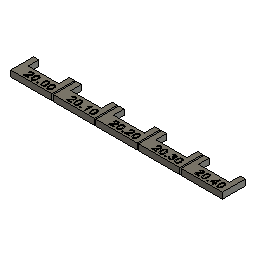
tolerance tester sloted v2 (Autodesk Fusion 360 design; units mm, degrees)
Autodesk Fusion 360 part; units mm, degrees
note: some values were not read from the file. Set by a fixed rule: which sketch regions a step uses.
sketch "Sketch1" plane through (0, 0, 0) normal (0, 1, 0) x (1, 0, 0)
  line L0 (0, 0) -> (27, 0)
  line L1 (27, 0) -> (27, -8)
  line L2 (27, -8) -> (0, -8)
  line L3 (0, -8) -> (0, 0)
  line L4 (27, 0) -> (0, 0)
  line L5 (0, 0) -> (0, 7)
  line L6 (27, 7) -> (27, 0)
  line L7 (13.5, 0) -> (13.5, 3.5)
  line L8 (3.5, 7) -> (3.5, 0)
  line L9 (3.5, 0) -> (23.5, 0)
  line L10 (23.5, 0) -> (23.5, 7)
  line L11 (23.5, 7) -> (3.5, 0) construction
  line L12 (3.5, 7) -> (23.5, 0) construction
  line L13 (0, 7) -> (3.5, 7)
  line L14 (23.5, 7) -> (27, 7)
  line L15 (51.5, 0) -> (51.4999, 7)
  line L16 (31.4, 0) -> (51.5, 0)
  line L17 (31.3999, 7) -> (31.4, 0)
  line L18 (27.9499, 0) -> (27.9499, 7)
  line L19 (27.9499, -8) -> (27.9499, 0)
  line L20 (27.9499, 0) -> (54.9499, 0)
  line L21 (54.9499, -8) -> (27.9499, -8)
  line L22 (54.9499, 0) -> (54.9499, -8)
  line L23 (27.9499, 7) -> (31.3999, 7)
  line L24 (54.9499, 7) -> (54.9499, 0)
  line L25 (54.9499, 0) -> (27.9499, 0)
  line L26 (51.4999, 7) -> (54.9499, 7)
  line L27 (55.8999, 7) -> (59.2999, 7)
  line L28 (107.5, 7) -> (110.85, 7)
  line L29 (55.8999, 0) -> (82.8999, 0)
  line L30 (79.4999, 0) -> (79.4999, 7)
  line L31 (83.85, -8) -> (83.85, 0)
  line L32 (59.2999, 0) -> (79.4999, 0)
  line L33 (59.2999, 7) -> (79.4999, 0) construction
  line L34 (59.2999, 7) -> (59.2999, 0)
  line L35 (69.3999, 0) -> (69.3999, 3.5)
  line L36 (79.4999, 7) -> (82.8999, 7)
  line L37 (82.8999, 0) -> (82.8999, -8)
  line L38 (107.5, 0) -> (107.5, 7)
  line L39 (87.2, 7) -> (87.2, 0)
  line L40 (55.8999, -8) -> (55.8999, 0)
  line L41 (87.2, 0) -> (107.5, 0)
  line L42 (110.85, 7) -> (110.85, 0)
  line L43 (82.8999, 0) -> (55.8999, 0)
  line L44 (107.5, 7) -> (87.2, 0) construction
  line L45 (83.85, 7) -> (87.2, 7)
  line L46 (110.85, 0) -> (83.85, 0)
  line L47 (110.85, -8) -> (83.85, -8)
  line L48 (83.85, 0) -> (83.85, 7)
  line L49 (79.4999, 7) -> (59.2999, 0) construction
  line L50 (82.8999, 7) -> (82.8999, 0)
  line L51 (97.35, 0) -> (97.35, 3.5)
  line L52 (55.8999, 0) -> (55.8999, 7)
  line L53 (83.85, 0) -> (110.85, 0)
  line L54 (110.85, 0) -> (110.85, -8)
  line L55 (87.2, 7) -> (107.5, 0) construction
  line L56 (82.8999, -8) -> (55.8999, -8)
  line L57 (7.0081, -6.0164) -> (18.0049, -5.9962) construction
  line L58 (18.0049, -5.9962) -> (17.9975, -1.9799) construction
  line L59 (17.9975, -1.9799) -> (7.0007, -2.0001) construction
  line L60 (7.0007, -2.0001) -> (7.0081, -6.0164) construction
  line L61 (7.0007, -2.0001) -> (135.5, -2.0001)
  line L62 (7.0081, -6.0164) -> (114.0079, -5.8204)
  line L63 (27.9499, -2.0001) -> (34.9499, -2.0001)
  line L64 (34.9499, -2.0001) -> (45.9489, -2.0001)
  line L65 (34.9544, -5.9574) -> (45.9521, -5.9451) construction
  line L66 (45.9521, -5.9451) -> (45.9477, -1.9877) construction
  line L67 (45.9477, -1.9877) -> (34.9499, -2.0001) construction
  line L68 (34.9499, -2.0001) -> (34.9544, -5.9574) construction
  line L69 (55.8999, -2.0001) -> (62.8999, -2.0001)
  line L70 (62.8999, -2.0001) -> (73.8899, -2.0001)
  line L71 (62.9041, -5.9057) -> (73.8932, -5.8939) construction
  line L72 (73.8932, -5.8939) -> (73.889, -1.9883) construction
  line L73 (73.889, -1.9883) -> (62.8999, -2.0001) construction
  line L74 (62.8999, -2.0001) -> (62.9041, -5.9057) construction
  line L75 (138.8, 0) -> (111.8, 0)
  line L76 (115.1, 0) -> (135.5, 0)
  line L77 (138.8, 7) -> (138.8, 0)
  line L78 (138.8, 0) -> (138.8, -8)
  line L79 (135.5, 0) -> (135.5, 7)
  line L80 (111.8, 0) -> (111.8, 7)
  line L81 (115.1, 7) -> (135.5, 0) construction
  line L82 (111.8, 7) -> (115.1, 7)
  line L83 (111.8, -8) -> (111.8, 0)
  line L84 (135.5, 7) -> (138.8, 7)
  line L85 (115.1, 7) -> (115.1, 0)
  line L86 (138.8, -8) -> (111.8, -8)
  line L87 (135.5, 7) -> (115.1, 0) construction
  line L88 (125.3, 0) -> (125.3, 3.5)
  line L89 (111.8, 0) -> (138.8, 0)
  line L90 (83.85, -2.0001) -> (90.85, -2.0001)
  line L91 (90.85, -2.0001) -> (101.84, -2.0001)
  line L92 (90.8533, -5.8525) -> (101.5332, -5.8432) construction
  line L93 (101.5332, -5.8432) -> (101.5299, -1.9908) construction
  line L94 (101.5299, -1.9908) -> (90.85, -2.0001) construction
  line L95 (90.85, -2.0001) -> (90.8533, -5.8525) construction
  line L96 (111.8, -2.0001) -> (118.8, -2.0001)
  line L97 (118.8, -2.0001) -> (129.79, -2.0001)
  line L98 (118.8001, -5.8199) -> (129.99, -5.8197) construction
  line L99 (129.99, -5.8197) -> (129.99, -1.9999) construction
  line L100 (129.99, -1.9999) -> (118.8, -2.0001) construction
  line L101 (118.8, -2.0001) -> (118.8001, -5.8199) construction
  point P0 (13.5, 3.5)
  point P1 (97.35, 3.5)
  point P2 (69.3999, 3.5)
  point P3 (125.3, 3.5)
  point P4 (142.0013, -5.9675)
  dimension "d55" = 27
  dimension "d56" = 8
  dimension "d57" = 27
  dimension "d58" = 7
  dimension "d59" = 3.5
  dimension "d60" = 20
  dimension "d61" = 27
  dimension "d62" = 8
  dimension "d63" = 27
  dimension "d64" = 7
  dimension "d66" = 20.1
  dimension "d67" = 27
  dimension "d68" = 8
  dimension "d69" = 27
  dimension "d70" = 7
  dimension "d71" = 3.5
  dimension "d72" = 20.2
  dimension "d73" = 27
  dimension "d74" = 8
  dimension "d75" = 27
  dimension "d76" = 7
  dimension "d77" = 3.5
  dimension "d78" = 20.3
  dimension "d79" = 4.7
  dimension "d80" = 107
  dimension "d81" = 7
  dimension "d82" = 10.999
  dimension "d83" = 4.7
  dimension "d84" = 7
  dimension "d85" = 10.99
  dimension "d86" = 4.6
  dimension "d87" = 27
  dimension "d88" = 8
  dimension "d89" = 27
  dimension "d90" = 7
  dimension "d91" = 3.5
  dimension "d92" = 20.4
  dimension "d93" = 7
  dimension "d94" = 10.99
  dimension "d95" = 4.6
  dimension "d96" = 7
  dimension "d97" = 10.99
  dimension "d98" = 4.6
  text T0 "20.00" font "Arial" height 4.7 align left top in box 10.9968 x 4.0163 at (7.0081, -6.0164) x (0.999998, 0.001832) y (-0.001832, 0.999998) spacing 1.14
  text T1 "20.10" font "Arial" height 4.7 align left top in box 10.9978 x 3.9573 at (34.9544, -5.9574) x (0.999999, 0.001122) y (-0.001122, 0.999999) spacing 1.14
  text T2 "20.20" font "Arial" height 4.6 align left top in box 10.9891 x 3.9056 at (62.9041, -5.9057) x (0.999999, 0.001074) y (-0.001074, 0.999999) spacing 1.14
  text T3 "20.30" font "Arial" height 4.6 align left top in box 10.6799 x 3.8524 at (90.8533, -5.8525) x (1, 0.000865) y (-0.000865, 1) spacing 1.14
  text T4 "20.40" font "Arial" height 4.6 align left top in box 11.19 x 3.8198 at (118.8001, -5.8199) x (1, 0.000014) y (-0.000014, 1) spacing 1.14
  constraint horizontal L0
  constraint vertical L1
  constraint horizontal L2
  constraint vertical L3
  constraint coincident L0.start L3.end
  constraint horizontal L4
  constraint vertical L5
  constraint horizontal L13
  constraint vertical L6
  constraint midpoint L4 L7.start
  constraint perpendicular L4 L7
  constraint parallel L8 L10
  constraint coincident L10.end L13
  constraint coincident L11 P0
  constraint coincident L12 P0
  constraint coincident P0 L7.end
  constraint collinear L13 L14
  constraint horizontal L20
  constraint vertical L22
  constraint horizontal L21
  constraint vertical L19
  constraint horizontal L25
  constraint vertical L18
  constraint horizontal L23
  constraint vertical L24
  constraint parallel L15 L17
  constraint coincident L15.end L23
  constraint collinear L23 L26
  constraint horizontal L29
  constraint vertical L37
  constraint horizontal L56
  constraint vertical L40
  constraint horizontal L43
  constraint vertical L52
  constraint horizontal L27
  constraint vertical L50
  constraint midpoint L35.start L43
  constraint perpendicular L35 L43
  constraint parallel L30 L34
  constraint coincident L30.end L27
  constraint coincident P2 L49
  constraint coincident P2 L33
  constraint coincident P2 L35.end
  constraint collinear L27 L36
  constraint horizontal L53
  constraint vertical L54
  constraint horizontal L47
  constraint vertical L31
  constraint horizontal L46
  constraint vertical L48
  constraint horizontal L45
  constraint vertical L42
  constraint midpoint L51.start L46
  constraint perpendicular L46 L51
  constraint parallel L38 L39
  constraint coincident L28.start L45
  constraint coincident P1 L44
  constraint coincident P1 L55
  constraint coincident P1 L51.end
  constraint collinear L28 L45
  constraint coincident L59.end
  constraint perpendicular L54 L61
  constraint coincident L57.start
  constraint perpendicular L60 L62
  constraint coincident L19 L63.start
  constraint coincident L61 L63.start
  constraint perpendicular L19 L63
  constraint parallel L61 L64
  constraint coincident L62
  constraint coincident L63.end
  constraint coincident L40 L69.start
  constraint coincident L61 L69.start
  constraint perpendicular L40 L69
  constraint parallel L61 L70
  constraint coincident L69.end
  constraint horizontal L89
  constraint vertical L78
  constraint horizontal L86
  constraint vertical L83
  constraint horizontal L75
  constraint vertical L80
  constraint horizontal L82
  constraint vertical L77
  constraint midpoint L88.start L75
  constraint perpendicular L75 L88
  constraint parallel L79 L85
  constraint coincident L79.end L82
  constraint coincident P3 L87
  constraint coincident P3 L81
  constraint coincident P3 L88.end
  constraint collinear L82 L84
  constraint coincident L31 L90.start
  constraint coincident L61 L90.start
  constraint perpendicular L31 L90
  constraint parallel L61 L91
  constraint coincident L90.end
  constraint coincident L83 L96.start
  constraint coincident L61 L96.start
  constraint perpendicular L83 L96
  constraint parallel L61 L97
  constraint coincident L96.end
  measures "d55" distance of L0.start L0.end
  measures "d56" distance of L0.start L2.end
  measures "d57" distance of L0.end L0.start
  measures "d58" distance of L0.end L6.start
  measures "d59" distance of L7.start P0
  measures "d60" distance of L8.end L9.end
  measures "d61" distance of L18.start L20.end
  measures "d62" distance of L18.start L19.start
  measures "d63" distance of L20.end L18.start
  measures "d64" distance of L20.end L24.start
  measures "d66" distance of L15.start L16.start
  measures "d67" distance of L29.start L29.end
  measures "d68" distance of L29.start L40.start
  measures "d69" distance of L29.end L29.start
  measures "d70" distance of L29.end L36.end
  measures "d71" distance of P2 L35.start
  measures "d72" distance of L30.start L32.start
  measures "d73" distance of L31.end L42.end
  measures "d74" distance of L31.end L31.start
  measures "d75" distance of L42.end L31.end
  measures "d76" distance of L28.end L42.end
  measures "d77" distance of L51.start P1
  measures "d78" distance of L38.start L39.end
  measures "d80" distance of L57.start L62.end
  measures "d81" distance of L63.start L63.end
  measures "d82" distance of L63.end L64.end
  measures "d84" distance of L69.start L69.end
  measures "d85" distance of L69.end L70.end
  measures "d87" distance of L75.end L75.start
  measures "d88" distance of L75.end L83.start
  measures "d89" distance of L75.end L75.start
  measures "d90" distance of L77.start L75.start
  measures "d91" distance of P3 L88.start
  measures "d92" distance of L76.end L76.start
  measures "d93" distance of L90.start L90.end
  measures "d94" distance of L90.end L91.end
  measures "d96" distance of L96.start L96.end
  measures "d97" distance of L96.end L97.end
extrude "Extrude1" add sketch "Sketch1" against normal blind 4 contours L0 L4 L5 L8 L13 | L0 L1 L2 L3 L4 L9 | L0 L4 L6 L10 L14 | L19 L21 L22 L62 | L19 L22 L61 L62 L63 L64 | L16 L19 L20 L22 L25 L61 L63 L64 | L17 L18 L20 L23 L25 | L37 L40 L56 L62 | L37 L40 L61 L62 L69 L70 | L15 L20 L24 L25 L26 | L29 L32 L37 L40 L43 L61 L69 L70 | L27 L29 L34 L43 L52 | L31 L47 L54 L62 | L31 L54 L61 L62 L90 L91 | L29 L30 L36 L43 L50 | L31 L41 L46 L53 L54 L61 L90 L91 | L39 L45 L46 L48 L53 | L75 L76 L78 L83 L86 L89 | L28 L38 L42 L46 L53 | L75 L80 L82 L85 L89 | L75 L77 L79 L84 L89 makes body 1 at (66.0333, 0, 5.3333) makes body 2 at (38.0999, 0, 5.3333) makes body 3 at (93.9666, 0, 5.3333) makes body 4 at (16.8333, 0, 5.3333) makes body 5 at (128.7, 0, 5.3333)
delete_face "DeleteFace1" 1 faces at (38.1, -1.3333, 0) on bodies 2
extrude "Extrude2" cut sketch "Sketch1" against normal blind 1.5 text T0 T1 T2 T4 T3 bodies 1 2 3 4 5
chamfer "Chamfer1" distance 0.3 angle 45 20 edges at (59.2999, -4, -3.5) (79.4999, -4, -3.5) (81.1999, -4, -7) (57.5999, -4, -7) (51.5, -4, -3.5) (31.4, -4, -3.5) (29.6749, -4, -7) (53.2249, -4, -7) (23.5, -4, -3.5) (3.5, -4, -3.5) (25.25, -4, -7) (1.75, -4, -7) (115.1, -4, -3.5) (135.5, -4, -3.5) (113.45, -4, -7) (137.15, -4, -7) (87.2, -4, -3.5) (107.5, -4, -3.5) (109.175, -4, -7) (85.525, -4, -7) on bodies 1 2 3 4 5
named bodies: "20.20", "20.10", "20.30", "20.00", "20.40"
